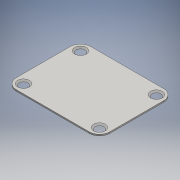
# Autodesk Inventor part: alguma parte da guitarra
Saved by Autodesk Inventor 2016 (Build 200138000, 138)
## iProperties
Created: 2018-10-30
Part Number: alguma parte da guitarra
Material: Genérico
Document SubType Name: Modeling
Designer: thiag
Density: 1 g/cm^3
Appearance: Padrão
Author: thiag
Autodesk Inventor part; units mm, degrees
ref_plane "YZ Plane" through (0, 0, 0) normal (1, 0, 0) x (0, 1, 0)
ref_plane "XZ Plane" through (0, 0, 0) normal (0, 1, 0) x (-1, 0, 0)
ref_plane "XY Plane" through (0, 0, 0) normal (0, 0, 1) x (1, 0, 0)
sketch "Esboço1" plane through (0, 0, 0) normal (0, 0, 1) x (1, 0, 0)
  line L0 (-26.8932, 18.2034) -> (37.1068, 18.2034)
  line L1 (37.1068, 18.2034) -> (37.1068, -32.7966)
  line L2 (37.1068, -32.7966) -> (-26.8932, -32.7966)
  line L3 (-26.8932, -32.7966) -> (-26.8932, 18.2034)
  circle A0 centre (-20.8932, 12.2034) radius 3
  circle A1 centre (-20.8932, -26.7966) radius 3
  circle A2 centre (31.1068, -26.7966) radius 3
  circle A3 centre (31.1068, 12.2034) radius 3
  dimension "d9" = 64
  dimension "d10" = 51
  dimension "d15" = 6
  dimension "d16" = 6
  dimension "d17" = 6
  dimension "d18" = 6
  constraints: 8 end point, 4 centre point, 2 parallel, 1 horizontal, 1 perpendicular
  measures "d9" distance of L1.end L2.end
  measures "d10" distance of L0.end L1.end
  measures "d15" diameter of A0
  measures "d16" diameter of A1
  measures "d17" diameter of A2
  measures "d18" diameter of A3
extrude "Extrusão1" add sketch "Esboço1" along normal blind 1
chamfer "Chanfro1" distance 1 angle 45 4 edges at (-23.8932, -26.7966, 1) (-23.8932, 12.2034, 1) (28.1068, 12.2034, 1) (28.1068, -26.7966, 1)
fillet "Arredondamento2" radius 7 4 edges at (-26.8932, -32.7966, 0.5) (37.1068, -32.7966, 0.5) (37.1068, 18.2034, 0.5) (-26.8932, 18.2034, 0.5)
